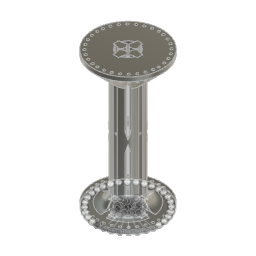
electrically_isolated_longerversion v13 (Autodesk Fusion 360 design; units mm, degrees)
Autodesk Fusion 360 part; units mm, degrees
sketch "Sketch1" plane through (0, 0, 0) normal (0, 0, 1) x (1, 0, 0)
  circle A0 centre (0, 0) radius 10
  circle A1 centre (0, 0) radius 2 construction
  line L0 (-10, 0) -> (10, 0) construction
  line L1 (-10, 0) -> (10, 0) construction
  line L2 (0, 10) -> (0, -10) construction
  line L3 (2, 0) -> (2, 9.798) construction
  line L4 (3.8, 3.2311) -> (3.8, -3.231) construction
  line L5 (3.8, 9.2499) -> (3.8, 0) construction
  spline S0 degree 5 poles (3.8, 3.2311) (3.6635, 3.1018) (3.4023, 2.8433) (3.0464, 2.4556) (2.6446, 1.9386) (2.2717, 1.2924) (2.0398, 0.6462) (1.9604, 0) (2.0398, -0.6462) (2.2717, -1.2924) (2.6446, -1.9386) (3.0464, -2.4556) (3.4023, -2.8433) (3.6635, -3.1018) (3.8, -3.231) knots 0 0 0 0 0 0 0.1 0.2 0.3 0.4 0.5 0.6 0.7 0.8 0.9 1 1 1 1 1 1
  line L6 (7.8, 2) -> (7.8, -2)
  line L7 (5.3, 2.5) -> (5.3, -2.5) construction
  line L8 (5.3, 8.48) -> (5.3, -8.48) construction
  spline S1 degree 5 poles (3.8, 3.2311) (3.8518, 3.1941) (3.9579, 3.1214) (4.1248, 3.0156) (4.3628, 2.8813) (4.6877, 2.7255) (5.0425, 2.5827) (5.4288, 2.4536) (5.8471, 2.3385) (6.2953, 2.2364) (6.7707, 2.1462) (7.1709, 2.0827) (7.4815, 2.0396) (7.6931, 2.0129) (7.8, 2) knots 0 0 0 0 0 0 0.1 0.2 0.3 0.4 0.5 0.6 0.7 0.8 0.9 1 1 1 1 1 1
  spline S2 degree 5 poles (3.8, -3.231) (3.8518, -3.1941) (3.9579, -3.1214) (4.1248, -3.0156) (4.3628, -2.8813) (4.6877, -2.7255) (5.0425, -2.5827) (5.4288, -2.4536) (5.8471, -2.3385) (6.2953, -2.2364) (6.7707, -2.1462) (7.1709, -2.0827) (7.4815, -2.0396) (7.6931, -2.0129) (7.8, -2) knots 0 0 0 0 0 0 0.1 0.2 0.3 0.4 0.5 0.6 0.7 0.8 0.9 1 1 1 1 1 1
  circle A2 centre (0, 0) radius 25
  line L9 (0, -25) -> (0, 25) construction
  circle A3 centre (0, 0) radius 22.5 construction
  circle A4 centre (0, -22.5) radius 0.85
  line L10 (11.8, 2) -> (11.8, -2)
  line L11 (11.8, -2) -> (7.8, -2)
  line L12 (11.8, 2) -> (7.8, 2)
  circle A5 centre (0, 0) radius 7.5
  spline S3 degree 5 poles (-3.2311, 3.8) (-3.1018, 3.6635) (-2.8433, 3.4023) (-2.4556, 3.0464) (-1.9386, 2.6446) (-1.2924, 2.2717) (-0.6462, 2.0398) (0, 1.9604) (0.6462, 2.0398) (1.2924, 2.2717) (1.9386, 2.6446) (2.4556, 3.0464) (2.8433, 3.4023) (3.1018, 3.6635) (3.231, 3.8) knots 0 0 0 0 0 0 0.1 0.2 0.3 0.4 0.5 0.6 0.7 0.8 0.9 1 1 1 1 1 1
  spline S4 degree 5 poles (3.231, 3.8) (3.1941, 3.8518) (3.1214, 3.9579) (3.0156, 4.1248) (2.8813, 4.3628) (2.7255, 4.6877) (2.5827, 5.0425) (2.4536, 5.4288) (2.3385, 5.8471) (2.2364, 6.2953) (2.1462, 6.7707) (2.0827, 7.1709) (2.0396, 7.4815) (2.0129, 7.6931) (2, 7.8) knots 0 0 0 0 0 0 0.1 0.2 0.3 0.4 0.5 0.6 0.7 0.8 0.9 1 1 1 1 1 1
  line L13 (2, 11.8) -> (2, 7.8)
  line L14 (-2, 11.8) -> (2, 11.8)
  line L15 (-2, 7.8) -> (2, 7.8)
  spline S5 degree 5 poles (-3.2311, 3.8) (-3.1941, 3.8518) (-3.1214, 3.9579) (-3.0156, 4.1248) (-2.8813, 4.3628) (-2.7255, 4.6877) (-2.5827, 5.0425) (-2.4536, 5.4288) (-2.3385, 5.8471) (-2.2364, 6.2953) (-2.1462, 6.7707) (-2.0827, 7.1709) (-2.0396, 7.4815) (-2.0129, 7.6931) (-2, 7.8) knots 0 0 0 0 0 0 0.1 0.2 0.3 0.4 0.5 0.6 0.7 0.8 0.9 1 1 1 1 1 1
  line L16 (-2, 11.8) -> (-2, 7.8)
  spline S6 degree 5 poles (-3.8, -3.2311) (-3.6635, -3.1018) (-3.4023, -2.8433) (-3.0464, -2.4556) (-2.6446, -1.9386) (-2.2717, -1.2924) (-2.0398, -0.6462) (-1.9604, 0) (-2.0398, 0.6462) (-2.2717, 1.2924) (-2.6446, 1.9386) (-3.0464, 2.4556) (-3.4023, 2.8433) (-3.6635, 3.1018) (-3.8, 3.231) knots 0 0 0 0 0 0 0.1 0.2 0.3 0.4 0.5 0.6 0.7 0.8 0.9 1 1 1 1 1 1
  spline S7 degree 5 poles (-3.8, 3.231) (-3.8518, 3.1941) (-3.9579, 3.1214) (-4.1248, 3.0156) (-4.3628, 2.8813) (-4.6877, 2.7255) (-5.0425, 2.5827) (-5.4288, 2.4536) (-5.8471, 2.3385) (-6.2953, 2.2364) (-6.7707, 2.1462) (-7.1709, 2.0827) (-7.4815, 2.0396) (-7.6931, 2.0129) (-7.8, 2) knots 0 0 0 0 0 0 0.1 0.2 0.3 0.4 0.5 0.6 0.7 0.8 0.9 1 1 1 1 1 1
  line L17 (-11.8, 2) -> (-7.8, 2)
  line L18 (-11.8, -2) -> (-11.8, 2)
  line L19 (-7.8, -2) -> (-7.8, 2)
  spline S8 degree 5 poles (-3.8, -3.2311) (-3.8518, -3.1941) (-3.9579, -3.1214) (-4.1248, -3.0156) (-4.3628, -2.8813) (-4.6877, -2.7255) (-5.0425, -2.5827) (-5.4288, -2.4536) (-5.8471, -2.3385) (-6.2953, -2.2364) (-6.7707, -2.1462) (-7.1709, -2.0827) (-7.4815, -2.0396) (-7.6931, -2.0129) (-7.8, -2) knots 0 0 0 0 0 0 0.1 0.2 0.3 0.4 0.5 0.6 0.7 0.8 0.9 1 1 1 1 1 1
  line L20 (-11.8, -2) -> (-7.8, -2)
  spline S9 degree 5 poles (3.2311, -3.8) (3.1018, -3.6635) (2.8433, -3.4023) (2.4556, -3.0464) (1.9386, -2.6446) (1.2924, -2.2717) (0.6462, -2.0398) (0, -1.9604) (-0.6462, -2.0398) (-1.2924, -2.2717) (-1.9386, -2.6446) (-2.4556, -3.0464) (-2.8433, -3.4023) (-3.1018, -3.6635) (-3.231, -3.8) knots 0 0 0 0 0 0 0.1 0.2 0.3 0.4 0.5 0.6 0.7 0.8 0.9 1 1 1 1 1 1
  spline S10 degree 5 poles (-3.231, -3.8) (-3.1941, -3.8518) (-3.1214, -3.9579) (-3.0156, -4.1248) (-2.8813, -4.3628) (-2.7255, -4.6877) (-2.5827, -5.0425) (-2.4536, -5.4288) (-2.3385, -5.8471) (-2.2364, -6.2953) (-2.1462, -6.7707) (-2.0827, -7.1709) (-2.0396, -7.4815) (-2.0129, -7.6931) (-2, -7.8) knots 0 0 0 0 0 0 0.1 0.2 0.3 0.4 0.5 0.6 0.7 0.8 0.9 1 1 1 1 1 1
  line L21 (-2, -11.8) -> (-2, -7.8)
  line L22 (2, -11.8) -> (-2, -11.8)
  line L23 (2, -7.8) -> (-2, -7.8)
  spline S11 degree 5 poles (3.2311, -3.8) (3.1941, -3.8518) (3.1214, -3.9579) (3.0156, -4.1248) (2.8813, -4.3628) (2.7255, -4.6877) (2.5827, -5.0425) (2.4536, -5.4288) (2.3385, -5.8471) (2.2364, -6.2953) (2.1462, -6.7707) (2.0827, -7.1709) (2.0396, -7.4815) (2.0129, -7.6931) (2, -7.8) knots 0 0 0 0 0 0 0.1 0.2 0.3 0.4 0.5 0.6 0.7 0.8 0.9 1 1 1 1 1 1
  line L24 (2, -11.8) -> (2, -7.8)
  circle A6 centre (22.5, 0) radius 0.85
  circle A7 centre (0, 22.5) radius 0.85
  circle A8 centre (-22.5, 0) radius 0.85
  circle A9 centre (4.4774, -22.05) radius 0.8625
  circle A10 centre (8.7758, -20.718) radius 0.875
  circle A11 centre (12.7231, -18.5573) radius 0.8875
  circle A12 centre (16.1615, -15.6543) radius 0.9
  circle A13 centre (18.9534, -12.1251) radius 0.9125
  line L25 (0, 0) -> (4.4774, -22.05) construction
  line L26 (0, 0) -> (8.7758, -20.718) construction
  line L27 (0, 0) -> (12.7231, -18.5573) construction
  line L28 (0, 0) -> (16.1615, -15.6543) construction
  line L29 (0, 0) -> (18.9534, -12.1251) construction
  circle A14 centre (20.9872, -8.1109) radius 0.925
  circle A15 centre (22.1815, -3.7723) radius 0.9375
  line L30 (20.9872, -8.1109) -> (0, 0) construction
  line L31 (22.1815, -3.7723) -> (0, 0) construction
  circle A16 centre (22.05, 4.4774) radius 0.8625
  circle A17 centre (20.718, 8.7758) radius 0.875
  circle A18 centre (18.5573, 12.7231) radius 0.8875
  circle A19 centre (15.6543, 16.1615) radius 0.9
  circle A20 centre (12.1251, 18.9534) radius 0.9125
  circle A21 centre (8.1109, 20.9872) radius 0.925
  circle A22 centre (3.7723, 22.1815) radius 0.9375
  circle A23 centre (-4.4774, 22.05) radius 0.8625
  circle A24 centre (-8.7758, 20.718) radius 0.875
  circle A25 centre (-12.7231, 18.5573) radius 0.8875
  circle A26 centre (-16.1615, 15.6543) radius 0.9
  circle A27 centre (-18.9534, 12.1251) radius 0.9125
  circle A28 centre (-20.9872, 8.1109) radius 0.925
  circle A29 centre (-22.1815, 3.7723) radius 0.9375
  circle A30 centre (-22.05, -4.4774) radius 0.8625
  circle A31 centre (-20.718, -8.7758) radius 0.875
  circle A32 centre (-18.5573, -12.7231) radius 0.8875
  circle A33 centre (-15.6543, -16.1615) radius 0.9
  circle A34 centre (-12.1251, -18.9534) radius 0.9125
  circle A35 centre (-8.1109, -20.9872) radius 0.925
  circle A36 centre (-3.7723, -22.1815) radius 0.9375
  line L32 (-8.8, 2) -> (-8.8, -2)
  line L33 (-2, -8.8) -> (2, -8.8)
  line L34 (8.8, -2) -> (8.8, 2)
  line L35 (2, 8.8) -> (-2, 8.8)
  point P0 (5.3, 0)
  point P1 (0, -22.5)
  point P2 (7.8, 0)
  point P3 (0, 2)
  point P4 (2.5, 5.3)
  point P5 (-2.5, 5.3)
  point P6 (-2, 0)
  point P7 (-5.3, 2.5)
  point P8 (-5.3, -2.5)
  point P9 (0, -2)
  point P10 (-2.5, -5.3)
  point P11 (2.5, -5.3)
  dimension "d3" = 20
  dimension "d4" = 4
  dimension "d9" = 1.8
  dimension "d11" = 1.8
  dimension "d12" = 6.4621
  dimension "d16" = 5
  dimension "d17" = 4
  dimension "d18" = 2
  dimension "d19" = 1.5
  dimension "d20" = 50
  dimension "d21" = 45
  dimension "d22" = 1.7
  dimension "d25" = 4
  dimension "d26" = 2.5
  dimension "d28" = 15
  dimension "d31" = 360
  dimension "d33" = 360
  dimension "d102" = 1.725
  dimension "d103" = 1.75
  dimension "d104" = 1.775
  dimension "d105" = 1.8
  dimension "d106" = 1.825
  dimension "d121" = 4.5
  dimension "d123" = 4.5
  dimension "d124" = 4.5
  dimension "d125" = 4.5
  dimension "d126" = 4.5
  dimension "d127" = 4.5
  dimension "d128" = 4.5
  dimension "d129" = 1.85
  dimension "d130" = 1.875
  dimension "d132" = 360
  dimension "d190" = 1
  dimension "d192" = 360
  constraint coincident A0.centre A1.centre
  constraint concentric A0 A1
  constraint coincident A0 L0.start
  constraint coincident A0 L0.end
  constraint horizontal L0
  constraint coincident A0 L2.start
  constraint coincident A0 L2.end
  constraint perpendicular L1 L2
  constraint coincident L1 L3.start
  constraint coincident A1 L3.start
  constraint coincident A0 L3.end
  constraint perpendicular L1 L3
  constraint perpendicular L1 L4
  constraint coincident A0 L5.start
  constraint coincident L0 L5.end
  constraint perpendicular L0 L5
  constraint midpoint L4 L5.end
  constraint vertical L6
  constraint perpendicular L0 L7
  constraint coincident A0 L8.start
  constraint coincident A0 L8.end
  constraint perpendicular L0 L8
  constraint midpoint L8 P0
  constraint midpoint L7 P0
  constraint concentric A0 A2
  constraint coincident A2 L9.start
  constraint coincident A2 L9.end
  constraint vertical L9
  constraint collinear L2 L9
  constraint concentric A2 A3
  constraint coincident L9 P1
  constraint coincident A3 P1
  constraint coincident P1 A4.centre
  constraint midpoint L9 A0.centre
  constraint vertical L10
  constraint coincident L0 P2
  constraint midpoint L6 P2
  constraint horizontal L12
  constraint horizontal L11
  constraint concentric A3 A5
  constraint coincident A3 A9.centre
  constraint coincident A3 A10.centre
  constraint coincident A3 A11.centre
  constraint coincident A3 A12.centre
  constraint coincident A3 A13.centre
  constraint coincident A9.centre L25.end
  constraint coincident A10.centre L26.end
  constraint coincident A11.centre L27.end
  constraint coincident A12.centre L28.end
  constraint coincident A13.centre L29.end
  constraint coincident A3 A14.centre
  constraint coincident A3 A15.centre
  constraint coincident A14.centre L30.start
  constraint coincident A15.centre L31.start
  constraint coincident L20 L32.end
  constraint perpendicular L20 L32
  constraint coincident L17 L32.start
  measures "d3" diameter of A0
  measures "d4" diameter of A1
  measures "d9" distance of L3.start L4
  measures "d11" distance of L3 L5
  measures "d12" distance of L4.start L4.end
  measures "d16" distance of L7.start L7.end
  measures "d17" distance of L6.end L6.start
  measures "d18" horizontal distance of A0.centre L3.start
  measures "d19" distance of L4 L7
  measures "d20" diameter of A2
  measures "d21" diameter of A3
  measures "d22" diameter of A4
  measures "d25" distance of L6 L10
  measures "d26" distance of P0 P2
  measures "d28" diameter of A5
  measures "d102" diameter of A9
  measures "d103" diameter of A10
  measures "d104" diameter of A11
  measures "d105" diameter of A12
  measures "d106" diameter of A13
  measures "d121" distance of P1 A9.centre
  measures "d123" distance of A9.centre A10.centre
  measures "d124" distance of A10.centre A11.centre
  measures "d125" distance of A11.centre A12.centre
  measures "d126" distance of A12.centre A13.centre
  measures "d127" distance of A13.centre A14.centre
  measures "d128" distance of A14.centre A15.centre
  measures "d129" diameter of A14
  measures "d130" diameter of A15
  measures "d190" distance of L19 L32
extrude "Extrude1" add sketch "Sketch1" along normal blind 3 contours A0 L11 L12 L34 | A0 L10 L11 L12 | A0 L13 L16 L35 | A0 L13 L14 L16 | L6 L11 L12 L34 | A0 L21 L22 L24 | A0 L21 L24 L33 | L13 L15 L16 L35 | L21 L23 L24 L33 | A0 L17 L20 L32 | A0 L17 L18 L20 | L17 L19 L20 L32 | A2 | A9 | A10 | A11 | A12 | A13 | A14 | A15 | A16 | A17 | A18 | A19 | A20 | A21 | A22 | A23 | A24 | A25 | A26 | A27 | A28 | A29 | A30 | A31 | A32 | A33 | A34 | A35 | A36 makes body 1
sketch "Sketch2" plane through (0, 0, 3) normal (0, 0, 1) x (-1, 0, 0)
  arc A0 (9.798, 2) -> (2, 9.798) centre (0, 0) ccw
  line L0 (9.798, 2) -> (7.8, 2)
  line L1 (7.8, 2) -> (7.8, -2)
  line L2 (7.8, -2) -> (9.798, -2)
  arc A1 (2, -9.798) -> (9.798, -2) centre (0, 0) ccw
  line L3 (2, -9.798) -> (2, -7.8)
  line L4 (2, -7.8) -> (-2, -7.8)
  line L5 (-2, -7.8) -> (-2, -9.798)
  arc A2 (-9.798, -2) -> (-2, -9.798) centre (0, 0) ccw
  line L6 (-9.798, -2) -> (-7.8, -2)
  line L7 (-7.8, -2) -> (-7.8, 2)
  line L8 (-7.8, 2) -> (-9.798, 2)
  arc A3 (-2, 9.798) -> (-9.798, 2) centre (0, 0) ccw
  line L9 (-2, 9.798) -> (-2, 7.8)
  line L10 (-2, 7.8) -> (2, 7.8)
  line L11 (2, 7.8) -> (2, 9.798)
  circle A4 centre (0, -22.5) radius 0.85
  circle A5 centre (22.5, 0) radius 0.85
  circle A6 centre (0, 22.5) radius 0.85
  circle A7 centre (-22.5, 0) radius 0.85
  circle A8 centre (0, 0) radius 25
  circle A9 centre (0, 0) radius 19.5
  dimension "d36" = 39
  constraint concentric A0 A9
  measures "d36" diameter of A9
extrude "Extrude2" add sketch "Sketch1" along normal blind 100 separate body contours L6 S1 S2 A5 | A5 S4 L15 S5 | S0 S1 S2 A5 | A5 S10 L23 S11 | A5 S3 S4 S5 | A5 S9 S10 S11 | A5 S7 L19 S8 | A5 S6 S7 S8 makes body 2 at (2.4618, 3.0723, 59.5238) makes body 3 at (3.0723, -2.4618, 59.5238) makes body 4 at (-3.0723, 2.4618, 59.5238) makes body 5 at (-2.4618, -3.0723, 59.5238)
copy_body "Body->Comp1" bodies 2 removing the originals makes body 6 in component "rod1"
copy_body "Body->Comp2" bodies 3 removing the originals makes body 7 in component "rod2"
copy_body "Body->Comp3" bodies 4 removing the originals makes body 8 in component "rod3"
copy_body "Body->Comp4" bodies 5 removing the originals makes body 9 in component "rod4"
extrude "Extrude1'" add sketch "Sketch1" along normal blind 100 separate body contours A0 S1 L12 A5 S4 L13 | A0 S2 L11 A5 S11 L24 | A0 A5 S5 L16 S7 L17 | A0 A5 S8 L20 S10 L21 makes body 10 at (-4.3019, 9.0274, 66.6667) makes body 11 at (9.6891, 2.4743, 33.3333) makes body 12 at (-2.4743, -9.6891, 66.6667) makes body 13 at (9.6891, -2.4743, 66.6667) in component "Component"
combine "Combine1" operation add target body 13 tool bodies 12 11 1 10 in component "Component"
fillet "Fillet1" radius 8 1 edges at (-7.0711, -7.0711, 3) on bodies 13 in component "Component"
fillet "Fillet1" radius 8 3 edges at (7.0711, -7.0711, 3) (7.0711, 7.0711, 3) (-7.0711, 7.0711, 3) on bodies 13 in component "Component"
ref_plane "WorkPlane1" through (-5.899, 5.899, 100) normal (0, 0, 1) x (1, 0, 0)
sketch "Sketch3" plane through (-5.8903, 5.8903, 100) normal (0, 0, 1) x (1, 0, 0)
  arc A0 (7.8903, -23.7788) -> (23.7788, -7.8903) centre (5.8903, -5.8903) ccw
  arc A1 (-11.9982, -7.8903) -> (3.8903, -23.7788) centre (5.8903, -5.8903) ccw
  arc A2 (3.8903, 11.9982) -> (-11.9982, -3.8903) centre (5.8903, -5.8903) ccw
  arc A3 (23.7788, -3.8903) -> (7.8903, 11.9982) centre (5.8903, -5.8903) ccw
  point P0 (18.6182, -18.6182)
  point P1 (18.6182, 6.8376)
  point P2 (-6.8376, 6.8376)
  point P3 (-6.8376, -18.6182)
  constraint midpoint A0 P0
  constraint midpoint A3 P1
  constraint midpoint A2 P2
  constraint midpoint A1 P3
ref_plane "WorkPlane2" through (7.0711, -7.0711, 100) normal (0.707107, -0.707107, 0) x (0.707107, 0.707107, 0)
ref_plane "WorkPlane3" through (7.0711, 7.0711, 100) normal (0.707107, 0.707107, 0) x (-0.707107, 0.707107, 0)
ref_plane "WorkPlane4" through (-7.0711, 7.0711, 100) normal (-0.707107, 0.707107, 0) x (-0.707107, -0.707107, 0)
ref_plane "WorkPlane5" through (-7.0711, -7.0711, 100) normal (-0.707107, -0.707107, 0) x (0.707107, -0.707107, 0)
sketch "Sketch4" plane through (7.0711, -7.0711, 100) normal (0.707107, -0.707107, 0) x (0.707107, 0.707107, 0)
  line L0 (25, -100) -> (-25, -100)
  line L1 (-1.6, -89) -> (0, -94.5)
  line L2 (0, -94.5) -> (1.6, -89)
  line L3 (-1.6, -89) -> (1.6, -89) construction
  line L4 (0, 0) -> (0, -100) construction
  line L5 (-1.6, -59) -> (0, -53.5)
  line L6 (0, -53.5) -> (1.6, -59)
  line L7 (-1.6, -59) -> (1.6, -59) construction
  line L8 (0, -83.5) -> (0, -94.5) construction
  line L9 (0, -64.5) -> (0, -53.5) construction
  line L10 (-1.6, -89) -> (-1.6, -59)
  line L11 (1.6, -89) -> (1.6, -59)
  line L12 (0, -50.75) -> (-1.6, -45.25)
  line L13 (-1.6, -45.25) -> (0, -50.75)
  line L14 (0, -50.75) -> (1.6, -45.25)
  line L15 (1.6, -45.25) -> (1.6, -15.25)
  line L16 (1.6, -15.25) -> (0, -9.75)
  line L17 (0, -9.75) -> (-1.6, -15.25)
  line L18 (-1.6, -15.25) -> (-1.6, -45.25)
  line L19 (-1.6, -15.25) -> (1.6, -15.25) construction
  line L20 (-1.6, -45.25) -> (1.6, -45.25) construction
  point P0 (0, -100)
  point P1 (0, -45.25)
  dimension "d52" = 5.5
  dimension "d56" = 3.2
  dimension "d57" = 100
  dimension "d61" = 3.2
  dimension "d147" = 30
  dimension "d148" = 5.5
  dimension "d149" = 5.5
  dimension "d253" = 30
  dimension "d254" = 2.75
  dimension "d256" = 5.5
  dimension "d257" = 5.5
  dimension "d258" = 3.2
  constraint midpoint L0 P0
  constraint horizontal L3
  constraint coincident P0 L4.end
  constraint vertical L4
  constraint coincident L8.start L4
  constraint coincident L1.end L4
  constraint coincident L4 L9.start
  constraint coincident L4 L5.end
  constraint horizontal L7
  constraint midpoint L3 L8
  constraint midpoint L7 L9
  constraint coincident L4 L12.start
  constraint parallel L4 L15
  constraint coincident L4 L16.end
  constraint horizontal L20
  constraint horizontal L19
  constraint parallel L15 L18
  constraint midpoint L20 P1
  constraint coincident L4 P1
  measures "d52" distance of L0 L1.end
  measures "d56" distance of L1.start L2.end
  measures "d57" distance of L0 L4.start
  measures "d61" distance of L5.start L6.end
  measures "d147" distance of L3 L7
  measures "d148" distance of L5.end L7
  measures "d149" distance of L1.end L3
  measures "d253" distance of L19 L20
  measures "d254" distance of L5.end L12.start
  measures "d256" distance of L16.end L19
  measures "d257" distance of L12.start L20
  measures "d258" distance of L15 L18
extrude "Extrude2'" cut sketch "Sketch4" along normal blind -100 and the other way blind -10 bodies 13 in component "Component"
sketch "Sketch5" plane through (-5.8903, 5.8903, 100) normal (0, 0, 1) x (1, 0, 0)
  circle A0 centre (5.8903, -5.8903) radius 25
  circle A1 centre (5.8903, -5.8903) radius 22.5 construction
  line L0 (5.8903, -30.8903) -> (5.8903, 19.1097) construction
  circle A2 centre (5.8903, -5.8903) radius 10
  line L1 (-4.1097, -5.8903) -> (15.8903, -5.8903)
  spline S0 degree 5 poles (2.6592, -2.0903) (2.6962, -2.0385) (2.7689, -1.9324) (2.8747, -1.7655) (3.009, -1.5275) (3.1648, -1.2025) (3.3076, -0.8478) (3.4367, -0.4615) (3.5518, -0.0432) (3.6539, 0.405) (3.7441, 0.8804) (3.8076, 1.2806) (3.8507, 1.5912) (3.8774, 1.8028) (3.8903, 1.9097) knots 0 0 0 0 0 0 0.1 0.2 0.3 0.4 0.5 0.6 0.7 0.8 0.9 1 1 1 1 1 1
  spline S1 degree 5 poles (2.6592, -2.0903) (2.7885, -2.2268) (3.047, -2.4879) (3.4347, -2.8439) (3.9517, -3.2457) (4.5979, -3.6186) (5.2441, -3.8505) (5.8903, -3.9299) (6.5365, -3.8505) (7.1827, -3.6186) (7.8289, -3.2457) (8.3459, -2.8439) (8.7336, -2.4879) (8.9921, -2.2268) (9.1213, -2.0903) knots 0 0 0 0 0 0 0.1 0.2 0.3 0.4 0.5 0.6 0.7 0.8 0.9 1 1 1 1 1 1
  spline S2 degree 5 poles (2.0903, -9.1213) (2.2268, -8.9921) (2.4879, -8.7336) (2.8439, -8.3459) (3.2457, -7.8289) (3.6186, -7.1827) (3.8505, -6.5365) (3.9299, -5.8903) (3.8505, -5.2441) (3.6186, -4.5979) (3.2457, -3.9517) (2.8439, -3.4347) (2.4879, -3.047) (2.2268, -2.7885) (2.0903, -2.6592) knots 0 0 0 0 0 0 0.1 0.2 0.3 0.4 0.5 0.6 0.7 0.8 0.9 1 1 1 1 1 1
  spline S3 degree 5 poles (9.6903, -2.6592) (9.5538, -2.7885) (9.2926, -3.047) (8.9367, -3.4347) (8.5349, -3.9517) (8.162, -4.5979) (7.9301, -5.2441) (7.8507, -5.8903) (7.9301, -6.5365) (8.162, -7.1827) (8.5349, -7.8289) (8.9367, -8.3459) (9.2926, -8.7336) (9.5538, -8.9921) (9.6903, -9.1213) knots 0 0 0 0 0 0 0.1 0.2 0.3 0.4 0.5 0.6 0.7 0.8 0.9 1 1 1 1 1 1
  circle A3 centre (5.8903, -5.8903) radius 2
  spline S4 degree 5 poles (9.1213, -9.6903) (8.9921, -9.5538) (8.7336, -9.2926) (8.3459, -8.9367) (7.8289, -8.5349) (7.1827, -8.162) (6.5365, -7.9301) (5.8903, -7.8507) (5.2441, -7.9301) (4.5979, -8.162) (3.9517, -8.5349) (3.4347, -8.9367) (3.047, -9.2926) (2.7885, -9.5538) (2.6592, -9.6903) knots 0 0 0 0 0 0 0.1 0.2 0.3 0.4 0.5 0.6 0.7 0.8 0.9 1 1 1 1 1 1
  spline S5 degree 5 poles (2.6592, -9.6903) (2.6962, -9.7421) (2.7689, -9.8482) (2.8747, -10.0151) (3.009, -10.253) (3.1648, -10.578) (3.3076, -10.9327) (3.4367, -11.3191) (3.5518, -11.7374) (3.6539, -12.1856) (3.7441, -12.661) (3.8076, -13.0612) (3.8507, -13.3718) (3.8774, -13.5834) (3.8903, -13.6903) knots 0 0 0 0 0 0 0.1 0.2 0.3 0.4 0.5 0.6 0.7 0.8 0.9 1 1 1 1 1 1
  line L2 (3.8903, -17.6903) -> (3.8903, -13.6903)
  line L3 (7.8903, -17.6903) -> (3.8903, -17.6903)
  line L4 (7.8903, -17.6903) -> (7.8903, -13.6903)
  spline S6 degree 5 poles (9.1213, -9.6903) (9.0844, -9.7421) (9.0117, -9.8482) (8.9059, -10.0151) (8.7716, -10.253) (8.6158, -10.578) (8.4729, -10.9327) (8.3439, -11.3191) (8.2288, -11.7374) (8.1267, -12.1856) (8.0365, -12.661) (7.973, -13.0612) (7.9299, -13.3718) (7.9032, -13.5834) (7.8903, -13.6903) knots 0 0 0 0 0 0 0.1 0.2 0.3 0.4 0.5 0.6 0.7 0.8 0.9 1 1 1 1 1 1
  circle A4 centre (5.8903, -5.8903) radius 7.5
  spline S7 degree 5 poles (9.1213, -2.0903) (9.0844, -2.0385) (9.0117, -1.9324) (8.9059, -1.7655) (8.7716, -1.5275) (8.6158, -1.2025) (8.4729, -0.8478) (8.3439, -0.4615) (8.2288, -0.0432) (8.1267, 0.405) (8.0365, 0.8804) (7.973, 1.2806) (7.9299, 1.5912) (7.9032, 1.8028) (7.8903, 1.9097) knots 0 0 0 0 0 0 0.1 0.2 0.3 0.4 0.5 0.6 0.7 0.8 0.9 1 1 1 1 1 1
  line L5 (3.8903, 5.9097) -> (7.8903, 5.9097)
  line L6 (3.8903, 5.9097) -> (3.8903, 1.9097)
  line L7 (3.8903, 1.9097) -> (7.8903, 1.9097)
  line L8 (7.8903, 5.9097) -> (7.8903, 1.9097)
  line L9 (-5.9097, -3.8903) -> (-1.9097, -3.8903)
  spline S8 degree 5 poles (2.0903, -2.6592) (2.0385, -2.6962) (1.9324, -2.7689) (1.7655, -2.8747) (1.5275, -3.009) (1.2025, -3.1648) (0.8478, -3.3076) (0.4615, -3.4367) (0.0432, -3.5518) (-0.405, -3.6539) (-0.8804, -3.7441) (-1.2806, -3.8076) (-1.5912, -3.8507) (-1.8028, -3.8774) (-1.9097, -3.8903) knots 0 0 0 0 0 0 0.1 0.2 0.3 0.4 0.5 0.6 0.7 0.8 0.9 1 1 1 1 1 1
  spline S9 degree 5 poles (2.0903, -9.1213) (2.0385, -9.0844) (1.9324, -9.0117) (1.7655, -8.9059) (1.5275, -8.7716) (1.2025, -8.6158) (0.8478, -8.4729) (0.4615, -8.3439) (0.0432, -8.2288) (-0.405, -8.1267) (-0.8804, -8.0365) (-1.2806, -7.973) (-1.5912, -7.9299) (-1.8028, -7.9032) (-1.9097, -7.8903) knots 0 0 0 0 0 0 0.1 0.2 0.3 0.4 0.5 0.6 0.7 0.8 0.9 1 1 1 1 1 1
  line L10 (-5.9097, -7.8903) -> (-1.9097, -7.8903)
  line L11 (-5.9097, -7.8903) -> (-5.9097, -3.8903)
  line L12 (-1.9097, -7.8903) -> (-1.9097, -3.8903)
  spline S10 degree 5 poles (9.6903, -2.6592) (9.7421, -2.6962) (9.8482, -2.7689) (10.0151, -2.8747) (10.253, -3.009) (10.578, -3.1648) (10.9327, -3.3076) (11.3191, -3.4367) (11.7374, -3.5518) (12.1856, -3.6539) (12.661, -3.7441) (13.0612, -3.8076) (13.3718, -3.8507) (13.5834, -3.8774) (13.6903, -3.8903) knots 0 0 0 0 0 0 0.1 0.2 0.3 0.4 0.5 0.6 0.7 0.8 0.9 1 1 1 1 1 1
  spline S11 degree 5 poles (9.6903, -9.1213) (9.7421, -9.0844) (9.8482, -9.0117) (10.0151, -8.9059) (10.253, -8.7716) (10.578, -8.6158) (10.9327, -8.4729) (11.3191, -8.3439) (11.7374, -8.2288) (12.1856, -8.1267) (12.661, -8.0365) (13.0612, -7.973) (13.3718, -7.9299) (13.5834, -7.9032) (13.6903, -7.8903) knots 0 0 0 0 0 0 0.1 0.2 0.3 0.4 0.5 0.6 0.7 0.8 0.9 1 1 1 1 1 1
  line L13 (17.6903, -7.8903) -> (13.6903, -7.8903)
  line L14 (17.6903, -3.8903) -> (13.6903, -3.8903)
  line L15 (13.6903, -3.8903) -> (13.6903, -7.8903)
  line L16 (17.6903, -3.8903) -> (17.6903, -7.8903)
  line L17 (7.8903, -13.6903) -> (3.8903, -13.6903)
  line L18 (9.6903, -2.6592) -> (9.6903, -9.1213)
  line L19 (11.1903, 2.5897) -> (11.1903, -14.3703)
  line L20 (7.8903, -5.8903) -> (7.8903, 3.9077)
  circle A5 centre (5.8903, -28.3903) radius 0.8
  circle A6 centre (-16.6097, -5.8903) radius 0.8
  circle A7 centre (28.3903, -5.8903) radius 0.8
  circle A8 centre (5.8903, 16.6097) radius 0.8
  point P0 (5.8903, 16.6097)
  point P1 (-16.6097, -5.8903)
  point P2 (5.8903, -28.3903)
  point P3 (28.3903, -5.8903)
  point P4 (11.1903, -14.3703)
  point P5 (5.8903, -7.8903)
  point P6 (8.3903, -11.1903)
  point P7 (11.1903, -3.3903)
  point P8 (11.1903, -8.3903)
  dimension "d77" = 1.6
  dimension "d78" = 1.6
  dimension "d79" = 1.6
  dimension "d80" = 1.6
  constraint coincident P2 A5.centre
  constraint coincident P1 A6.centre
  constraint coincident P3 A7.centre
  constraint coincident P0 A8.centre
  measures "d77" diameter of A5
  measures "d78" diameter of A6
  measures "d79" diameter of A7
  measures "d80" diameter of A8
sketch "Sketch6" plane through (-7.0711, -7.0711, 100) normal (-0.707107, -0.707107, 0) x (0.707107, -0.707107, 0)
  line L0 (25, -100) -> (-25, -100)
  line L1 (0, -100) -> (0, 0) construction
  line L2 (0, -94.5) -> (-1.6, -89)
  line L3 (1.6, -89) -> (0, -94.5)
  line L4 (-1.6, -59) -> (0, -53.5)
  line L5 (0, -53.5) -> (1.6, -59)
  line L6 (0, -53.5) -> (0, -64.5) construction
  line L7 (-1.6, -59) -> (1.6, -59) construction
  line L8 (-1.6, -89) -> (1.6, -89) construction
  line L9 (0, -83.5) -> (0, -94.5) construction
  line L10 (1.6, -89) -> (1.6, -59)
  line L11 (-1.6, -59) -> (-1.6, -89)
  line L12 (0, -50.75) -> (-1.6, -45.25)
  line L13 (-1.6, -45.25) -> (-1.6, -15.25)
  line L14 (-1.6, -15.25) -> (0, -9.75)
  line L15 (0, -9.75) -> (1.6, -15.25)
  line L16 (1.6, -45.25) -> (0, -50.75)
  line L17 (-1.6, -45.25) -> (1.6, -45.25) construction
  line L18 (-1.6, -15.25) -> (1.6, -15.25) construction
  line L19 (1.6, -45.25) -> (1.6, -15.25)
  point P0 (0, -100)
  point P1 (0, -45.25)
  dimension "d62" = 100
  dimension "d63" = 5.5
  dimension "d67" = 3.2
  dimension "d150" = 5.5
  dimension "d151" = 5.5
  dimension "d152" = 30
  dimension "d259" = 2.75
  dimension "d260" = 3.2
  dimension "d261" = 5.5
  dimension "d262" = 5.5
  dimension "d263" = 30
  constraint midpoint L0 P0
  constraint coincident P0 L1.start
  constraint perpendicular L0 L1
  constraint coincident L1 L2.start
  constraint coincident L1 L9.start
  constraint coincident L1 L6.end
  constraint coincident L1 L4.end
  constraint perpendicular L6 L7
  constraint parallel L7 L8
  constraint midpoint L8 L9
  constraint midpoint L6 L7
  constraint perpendicular L7 L10
  constraint coincident L1 L12.start
  constraint coincident L1 L14.end
  constraint midpoint L17 P1
  constraint vertical L13
  constraint vertical L19
  constraint horizontal L17
  constraint horizontal L18
  constraint coincident L1 P1
  measures "d62" distance of P0 L1.end
  measures "d63" distance of P0 L2.start
  measures "d67" distance of L2.end L3.start
  measures "d150" distance of L2.start L8
  measures "d151" distance of L4.end L7
  measures "d152" distance of L7 L8
  measures "d259" distance of L4.end L12.start
  measures "d260" distance of L13 L19
  measures "d261" distance of L12.start L17
  measures "d262" distance of L14.end L18
  measures "d263" distance of L17 L18
extrude "Extrude3" cut sketch "Sketch6" along normal blind -100 and the other way blind -5 bodies 13 in component "Component"
extrude "Extrude4" add sketch "Sketch5" against normal blind 3 contours A0 | A2 L6 L7 L8 L20 | A2 L5 L6 L8 | A2 L13 L14 L16 | A2 L1 L14 L15 | A2 L1 L13 L15 | A2 L1 L9 L12 | A2 L9 L10 L11 | A2 L1 L10 L12 | A2 L2 L3 L4 | A2 L2 L4 L17 | A5 | A6 | A7 | A8 bodies 13 in component "Component"
chamfer "Chamfer1" distance 15 angle 45 1 edges at (-7.0711, 7.0711, 97) on bodies 13 in component "Component"
chamfer "Chamfer1" distance 15 angle 45 3 edges at (-7.0711, -7.0711, 97) (7.0711, -7.0711, 97) (7.0711, 7.0711, 97) on bodies 13 in component "Component"
combine "Combine1'" operation add target body 7 tool bodies 6 9 8 13 in component "rod2"
extrude "Extrude2''" cut sketch "Sketch5" against normal blind 100 contours S0 A4 L7 L20 | L1 A4 S10 L15 | L1 A4 S10 L19 | S1 A4 S7 L20 | L1 S10 L18 L19 | S0 S1 A4 L20 | L1 A4 S11 L15 | L1 A4 S11 L19 | L1 S3 L18 | L1 S11 L18 L19 | L1 A4 S8 L12 | L1 S3 L18 | L1 A4 S9 L12 | L1 S2 A4 S8 | L1 S2 A4 S9 | S4 S5 S6 A4 | S5 S6 A4 L17 bodies 7 in component "rod2"
extrude "Extrude1''" add sketch "Sketch5" against normal blind 100 separate body contours S0 A4 L7 L20 | A4 S7 L20 | L1 A4 S10 L15 | L1 A4 S10 L19 | S1 A4 S7 L20 | L1 S10 L18 L19 | S0 S1 A4 L20 | L1 A4 S11 L15 | L1 A4 S11 L19 | L1 S3 L18 | L1 S11 L18 L19 | L1 A4 S8 L12 | L1 S3 L18 | L1 A4 S9 L12 | L1 S2 A4 S8 | L1 S2 A4 S9 | S4 S5 S6 A4 | S5 S6 A4 L17 makes body 14 at (-7.8, -0.6667, 66.6667) makes body 15 at (-0.6667, 7.8, 66.6667) makes body 16 at (0.6667, -7.8, 66.6667) makes body 17 at (7.8, 0.6667, 66.6667) in component "Component'"
ref_plane "WorkPlane6" through (-17.6777, 17.6777, 1.5) normal (-0.707107, 0.707107, 0) x (-0.707107, -0.707107, 0)
sketch "Sketch7" plane through (-17.6777, 17.6777, 2) normal (-0.707107, 0.707107, 0) x (0.707107, 0.707107, 0)
  circle A0 centre (0, 0) radius 0.8
  dimension "d94" = 1.6
  constraint coincident A0.centre origin
  measures "d94" diameter of A0
extrude "Extrude3'" cut sketch "Sketch7" against normal blind 15 bodies 7 in component "rod2"
pattern_circular "C-Pattern1" count 4 over 360 about axis through (0, 0, 1.75) along (0, 0, 1) of "Extrude3'" in component "rod2"
extrude "Extrude2'''" cut sketch "Sketch1" along normal blind 1.6 contours L6 S1 S2 A5 | A5 S4 L15 S5 | S0 S1 S2 A5 | A5 S10 L23 S11 | A5 S3 S4 S5 | A5 S9 S10 S11 | A5 S7 L19 S8 | A5 S6 S7 S8 bodies 14 15 16 17 in component "Component'"
extrude "Extrude6" add sketch "Sketch1" along normal blind 1.6 contours L6 S1 S2 A5 | A5 S4 L15 S5 | S0 S1 S2 A5 | A5 S10 L23 S11 | A5 S3 S4 S5 | A5 S9 S10 S11 | A5 S7 L19 S8 | A5 S6 S7 S8 bodies 7 in component "rod2"
extrude "Extrude9" add sketch "Sketch5" against normal blind 3 contours A2 L6 L7 L8 L20 bodies 7 in component "rod2"
extrude "Extrude10" add 4 faces at (-0.044, -4.1114, 1.6) (-4.1114, 0.044, 1.6) (0.044, 4.1114, 1.6) (4.1114, -0.044, 1.6) along direction (0, 0, 1) blind 100 on bodies 7 bodies 7 in component "rod2"
extrude "Extrude11" cut 4 faces at (-0.044, -4.1114, 101.6) (-4.1114, 0.044, 101.6) (0.044, 4.1114, 101.6) (4.1114, -0.044, 101.6) along direction (0, 0, -1) blind 100 on bodies 7 bodies 7 in component "rod2"
extrude "Extrude12" add sketch "Sketch1" along normal blind 1.6 contours A0 L13 L16 L35 | A0 L13 L14 L16 | L13 L15 L16 L35 bodies 7 in component "rod2"
sketch "Sketch8" plane through (7.8, 0, 0) normal (1, 0, 0) x (0, 1, 0)
  line L0 (-2, 1.6) -> (2, 1.6)
  line L1 (2, 1.6) -> (2, 100)
  line L2 (2, 100) -> (-2, 100)
  line L3 (-2, 100) -> (-2, 1.6)
  line L4 (-2, 50.8) -> (2, 50.8) construction
  line L5 (0, 1.6) -> (0, 100) construction
  circle A0 centre (0, 50.8) radius 0.7
  dimension "d174" = 1.4
  constraint midpoint L3 L4.start
  constraint midpoint L1 L4.end
  constraint midpoint L0 L5.start
  constraint midpoint L2 L5.end
  constraint midpoint L4 A0.centre
  measures "d174" diameter of A0
extrude "Extrude4'" cut sketch "Sketch8" against normal blind 3.5 contours A0 bodies 17 in component "Component'"
sketch "Sketch9" plane through (0, -7.8, 0) normal (0, -1, 0) x (1, 0, 0)
  line L0 (-2, 1.6) -> (2, 1.6)
  line L1 (2, 1.6) -> (2, 100)
  line L2 (2, 100) -> (-2, 100)
  line L3 (-2, 100) -> (-2, 1.6)
  line L4 (0, 1.6) -> (0, 100) construction
  line L5 (-2, 50.8) -> (2, 50.8) construction
  circle A0 centre (0, 50.8) radius 0.7
  dimension "d181" = 1.4
  constraint midpoint L0 L4.start
  constraint midpoint L2 L4.end
  constraint midpoint L3 L5.start
  constraint midpoint L1 L5.end
  constraint midpoint L4 A0.centre
  measures "d181" diameter of A0
sketch "Sketch10" plane through (0, 7.8, 0) normal (0, 1, 0) x (-1, 0, 0)
  line L0 (-2, 1.6) -> (2, 1.6)
  line L1 (2, 100) -> (-2, 100)
  line L2 (-2, 100) -> (-2, 1.6)
  line L3 (0, 100) -> (0, 1.6) construction
  line L4 (-2, 50.8) -> (2, 50.8) construction
  circle A0 centre (0, 50.8) radius 0.7
  line L5 (2, 1.6) -> (2, 100)
  dimension "d182" = 1.4
  constraint midpoint L1 L3.start
  constraint midpoint L0 L3.end
  constraint midpoint L2 L4.start
  constraint midpoint L4 A0.centre
  measures "d182" diameter of A0
sketch "Sketch11" plane through (-7.8, 0, 0) normal (-1, 0, 0) x (0, -1, 0)
  line L0 (-2, 1.6) -> (2, 1.6)
  line L1 (2, 1.6) -> (2, 100)
  line L2 (2, 100) -> (-2, 100)
  line L3 (-2, 100) -> (-2, 1.6)
  line L4 (0, 100) -> (0, 1.6) construction
  line L5 (-2, 50.8) -> (2, 50.8) construction
  circle A0 centre (0, 50.8) radius 0.7
  dimension "d183" = 1.4
  constraint midpoint L2 L4.start
  constraint midpoint L0 L4.end
  constraint midpoint L3 L5.start
  constraint midpoint L1 L5.end
  constraint midpoint L4 A0.centre
  measures "d183" diameter of A0
extrude "Extrude5" cut sketch "Sketch9" against normal blind 3.5 contours A0 bodies 16 in component "Component'"
extrude "Extrude6'" cut sketch "Sketch10" against normal blind 3.5 contours A0 bodies 15 in component "Component'"
extrude "Extrude7" cut sketch "Sketch11" against normal blind 3.5 contours A0 bodies 14 in component "Component'"
extrude "Extrude13" cut sketch "Sketch1" along normal blind 110 contours L6 L11 L12 L34 | L13 L15 L16 L35 | L21 L23 L24 L33 | L17 L19 L20 L32 bodies 7 in component "rod2"
extrude "Extrude8" add sketch "Sketch1" along normal blind 100 contours L6 L11 L12 L34 | L13 L15 L16 L35 | L21 L23 L24 L33 | L17 L19 L20 L32 bodies 14 15 16 17 in component "Component'"
extrude "Extrude9'" cut sketch "Sketch1" along normal blind 1.6 contours L6 L11 L12 L34 | L13 L15 L16 L35 | L21 L23 L24 L33 | L17 L19 L20 L32 bodies 14 15 16 17 in component "Component'"
extrude "Extrude14" add sketch "Sketch1" along normal blind 1.6 contours L6 L11 L12 L34 | L13 L15 L16 L35 | L21 L23 L24 L33 | L17 L19 L20 L32 bodies 7 in component "rod2"
combine "Combine2" operation add target body 7 tool bodies 17 15 14 16 in component "rod2"
chamfer "Chamfer5" distance 15.99 angle 45 4 edges at (-8.8, 0, 97) (0, -8.8, 97) (8.8, 0, 97) (0, 8.8, 97) on bodies 7 in component "rod2"
extrude "Extrude5'" cut sketch "Sketch1" along normal blind 200 contours A4 | A6 | A7 | A8 | A9 | A10 | A11 | A12 | A13 | A14 | A15 | A16 | A17 | A18 | A19 | A20 | A21 | A22 | A23 | A24 | A25 | A26 | A27 | A28 | A29 | A30 | A31 | A32 | A33 | A34 | A35 | A36 bodies 7 in component "rod2"
extrude "Extrude15" cut sketch "Sketch1" along normal blind 100 contours L6 L11 L12 L34 | L13 L15 L16 L35 | L6 S1 S2 A5 | L21 L23 L24 L33 | A5 S4 L15 S5 | S0 S1 S2 A5 | A5 S10 L23 S11 | L17 L19 L20 L32 | A5 S3 S4 S5 | A5 S9 S10 S11 | A5 S7 L19 S8 | A5 S6 S7 S8 bodies 7 in component "rod2"
extrude "Extrude16" add sketch "Sketch1" along normal blind 1.6 contours L6 L11 L12 L34 | L13 L15 L16 L35 | L6 S1 S2 A5 | L21 L23 L24 L33 | A5 S4 L15 S5 | S0 S1 S2 A5 | A5 S10 L23 S11 | L17 L19 L20 L32 | A5 S3 S4 S5 | A5 S9 S10 S11 | A5 S7 L19 S8 | A5 S6 S7 S8 bodies 7 in component "rod2"
extrude "Extrude17" add 4 faces at (-4.111, 0.0345, 1.6) (-0.0345, -4.111, 1.6) (0.0345, 4.111, 1.6) (4.111, -0.0345, 1.6) along direction (0, 0, 1) blind 98.4 separate body on bodies 7 makes body 18 at (2.4618, 3.0723, 60.1714) makes body 19 at (-3.0723, 2.4618, 60.1714) makes body 20 at (-2.4618, -3.0723, 60.1714) makes body 21 at (3.0723, -2.4618, 60.1714) in component "rod2"
extrude "Extrude3''" add sketch "Sketch1" along normal blind 100 separate body contours L6 L11 L12 L34 | L13 L15 L16 L35 | L6 S1 S2 A5 | L21 L23 L24 L33 | A5 S4 L15 S5 | S0 S1 S2 A5 | A5 S10 L23 S11 | L17 L19 L20 L32 | A5 S3 S4 S5 | A5 S9 S10 S11 | A5 S7 L19 S8 | A5 S6 S7 S8 makes body 22 at (2.4618, 3.0723, 59.5238) makes body 23 at (3.0723, -2.4618, 59.5238) makes body 24 at (-3.0723, 2.4618, 59.5238) makes body 25 at (-2.4618, -3.0723, 59.5238)
copy_body "Body->Comp6" bodies 22 removing the originals makes body 26 in component "Component''"
copy_body "Body->Comp7" bodies 23 removing the originals makes body 27 in component "Component'''"
copy_body "Body->Comp8" bodies 24 removing the originals makes body 28 in component "Component''''"
copy_body "Body->Comp9" bodies 25 removing the originals makes body 29 in component "Component'''''"
extrude "Extrude1'''" cut sketch "Sketch1" along normal blind 1.6 contours L6 L11 L12 L34 | L13 L15 L16 L35 | L6 S1 S2 A5 | L21 L23 L24 L33 | A5 S4 L15 S5 | S0 S1 S2 A5 | A5 S10 L23 S11 | L17 L19 L20 L32 | A5 S3 S4 S5 | A5 S9 S10 S11 | A5 S7 L19 S8 | A5 S6 S7 S8 bodies 26 in component "Component''"
extrude "Extrude1''''" cut sketch "Sketch1" along normal blind 1.6 contours L6 L11 L12 L34 | L13 L15 L16 L35 | L6 S1 S2 A5 | L21 L23 L24 L33 | A5 S4 L15 S5 | S0 S1 S2 A5 | A5 S10 L23 S11 | L17 L19 L20 L32 | A5 S3 S4 S5 | A5 S9 S10 S11 | A5 S7 L19 S8 | A5 S6 S7 S8 bodies 27 in component "Component'''"
extrude "Extrude1'''''" cut sketch "Sketch1" along normal blind 1.6 contours L6 L11 L12 L34 | L13 L15 L16 L35 | L6 S1 S2 A5 | L21 L23 L24 L33 | A5 S4 L15 S5 | S0 S1 S2 A5 | A5 S10 L23 S11 | L17 L19 L20 L32 | A5 S3 S4 S5 | A5 S9 S10 S11 | A5 S7 L19 S8 | A5 S6 S7 S8 bodies 28 in component "Component''''"
extrude "Extrude1''''''" cut sketch "Sketch1" along normal blind 1.6 contours L6 L11 L12 L34 | L13 L15 L16 L35 | L6 S1 S2 A5 | L21 L23 L24 L33 | A5 S4 L15 S5 | S0 S1 S2 A5 | A5 S10 L23 S11 | L17 L19 L20 L32 | A5 S3 S4 S5 | A5 S9 S10 S11 | A5 S7 L19 S8 | A5 S6 S7 S8 bodies 29 in component "Component'''''"
extrude "Extrude18" cut 4 faces at (-0.0345, -4.111, 100) (-4.111, 0.0345, 100) (0.0345, 4.111, 100) (4.111, -0.0345, 100) along direction (0, 0, -1) blind 100 on bodies 18 19 20 21 bodies 7 18 19 20 21 in component "rod2"
extrude "Extrude19" add sketch "Sketch1" along normal blind 1.6 contours L6 L11 L12 L34 | L13 L15 L16 L35 | L6 S1 S2 A5 | L21 L23 L24 L33 | A5 S4 L15 S5 | S0 S1 S2 A5 | A5 S10 L23 S11 | L17 L19 L20 L32 | A5 S3 S4 S5 | A5 S9 S10 S11 | A5 S7 L19 S8 | A5 S6 S7 S8 bodies 7 18 19 20 21 in component "rod2"
extrude "Extrude2''''" [suppressed] in component "Component'''"
extrude "Extrude2'''''" cut sketch "Sketch11" along normal blind 1 and the other way blind 3 contours A0 bodies 28 in component "Component''''"
extrude "Extrude2''''''" cut sketch "Sketch10" along normal blind 1 and the other way blind 3 contours A0 bodies 26 in component "Component''"
extrude "Extrude2'''''''" cut sketch "Sketch9" along normal blind 1 and the other way blind 3 contours A0 bodies 29 in component "Component'''''"
extrude "Extrude3'''" cut sketch "Sketch8" along normal blind 1 and the other way blind 3 contours A0 bodies 27 in component "Component'''"
fillet "Fillet1'" radius 0.5 2 edges at (3.231, 3.8, 50.8) (-3.2311, 3.8, 50.8) on bodies 26 in component "Component''"
fillet "Fillet1''" radius 0.5 2 edges at (3.8, -3.231, 50.8) (3.8, 3.2311, 50.8) on bodies 27 in component "Component'''"
fillet "Fillet1'''" radius 0.5 2 edges at (-3.8, 3.231, 50.8) (-3.8, -3.2311, 50.8) on bodies 28 in component "Component''''"
fillet "Fillet1''''" radius 0.5 2 edges at (3.2311, -3.8, 50.8) (-3.231, -3.8, 50.8) on bodies 29 in component "Component'''''"
fillet "Fillet1'''''" radius 0.5 8 edges at (3.8, 3.2311, 0.8) (3.231, 3.8, 0.8) (3.8, -3.231, 0.8) (3.2311, -3.8, 0.8) (-3.231, -3.8, 0.8) (-3.8, -3.2311, 0.8) (-3.8, 3.231, 0.8) (-3.2311, 3.8, 0.8) on bodies 7 in component "rod2"
component "Component" placed x (1, 0, 0) y (0, 1, 0) z (0, 0, 1) at (0, 0, 0)
component "Component'" placed x (1, 0, 0) y (0, 1, 0) z (0, 0, 1) at (0, 0, 0)
component "rod1" placed x (1, 0, 0) y (0, 1, 0) z (0, 0, 1) at (0, 0, 0)
component "rod2" placed x (1, 0, 0) y (0, 1, 0) z (0, 0, 1) at (0, 0, 0)
component "rod3" placed x (1, 0, 0) y (0, 1, 0) z (0, 0, 1) at (0, 0, 0)
component "rod4" placed x (1, 0, 0) y (0, 1, 0) z (0, 0, 1) at (0, 0, 0)
component "Component'" placed x (1, 0, 0) y (0, 1, 0) z (0, 0, 1) at (0, 0, 0)
component "Component''" placed x (1, 0, 0) y (0, 1, 0) z (0, 0, 1) at (0, 0, 0)
component "Component'''" placed x (1, 0, 0) y (0, 1, 0) z (0, 0, 1) at (0, 0, 0)
component "Component''''" placed x (1, 0, 0) y (0, 1, 0) z (0, 0, 1) at (0, 0, 0)
component "Component'''''" placed x (1, 0, 0) y (0, 1, 0) z (0, 0, 1) at (0, 0, 0)
equation "r0 = 2 mm"
equation "quadrupole_diameter = 20 mm"
equation "d3 = quadrupole_diameter"
equation "d4 = r0 * 2"
equation "parabolic_width = 6.4621 mm"
equation "parabolic_height = 1.8 mm"
equation "d9 = parabolic_height"
equation "d11 = parabolic_height"
equation "d12 = parabolic_width"
equation "rod_length = 10 mm"
equation "d16 = r0 * 2.5"
equation "d17 = r0 * 2"
equation "d18 = r0"
equation "d19 = r0 * 0.75"
equation "d21 = outer_circle_diameter"
equation "diameter_outer_holes = 1.6 mm"
equation "outer_circle_diameter = 45 mm"
equation "quadrupole_inner_diameter = 15 mm"
equation "d28 = quadrupole_inner_diameter"
equation "d34 = baseplate_height"
equation "d36 = attachment_point_slope_start"
equation "attachment_point_slope_start = 39 mm"
equation "height = 100 mm"
equation "d39 = height"
equation "d41 = height"
equation "d44 = fillet_length"
equation "fillet_length = 8 mm"
equation "d47 = fillet_length"
equation "diamond_height = 30 mm"
equation "diamond_width = 3.2 mm"
equation "d52 = diamond_spacing"
equation "d56 = diamond_width"
equation "d57 = height"
equation "diamond_spacing = 5.5 mm"
equation "d61 = diamond_width"
equation "d62 = height"
equation "d63 = diamond_spacing"
equation "d67 = diamond_width"
equation "baseplate_height = 3 mm"
equation "d73 = -baseplate_height"
equation "d77 = diameter_outer_holes"
equation "d78 = diameter_outer_holes"
equation "d79 = diameter_outer_holes"
equation "d80 = diameter_outer_holes"
equation "d83 = ( outer_circle_diameter - quadrupole_inner_diameter ) / 2"
equation "d84 = ( outer_circle_diameter - quadrupole_inner_diameter ) / 2"
equation "chamfer_distance = 15 mm + 0.7979 mm"
equation "d89 = -height"
equation "d91 = -height"
equation "d94 = diameter_outer_holes"
equation "d121 = hole_spacing"
equation "hole_spacing = 4.5 mm"
equation "d123 = hole_spacing"
equation "d124 = hole_spacing"
equation "d125 = hole_spacing"
equation "d126 = hole_spacing"
equation "d127 = hole_spacing"
equation "d128 = hole_spacing"
equation "quadrupolerods_fillet = 0.4 mm"
equation "pla_bottom_conductive_base = 1.6 mm"
equation "d141 = pla_bottom_conductive_base"
equation "d143 = pla_bottom_conductive_base"
equation "d147 = diamond_height"
equation "d148 = diamond_spacing"
equation "d149 = diamond_spacing"
equation "d150 = diamond_spacing"
equation "d151 = diamond_spacing"
equation "d152 = diamond_height"
equation "d162 = -baseplate_height"
equation "d164 = height"
equation "d168 = -height"
equation "d172 = pla_bottom_conductive_base"
equation "d174 = wire_diam"
equation "wire_depth = 3.5 mm"
equation "wire_diam = 1.4 mm"
equation "d181 = wire_diam"
equation "d182 = wire_diam"
equation "d183 = wire_diam"
equation "d184 = -wire_depth"
equation "d186 = -wire_depth"
equation "d188 = -wire_depth"
equation "d193 = height + 10 mm"
equation "d195 = height"
equation "d197 = pla_bottom_conductive_base"
equation "d199 = pla_bottom_conductive_base"
equation "d202 = height"
equation "d204 = pla_bottom_conductive_base"
equation "d206 = height - pla_bottom_conductive_base"
equation "d208 = height"
equation "d210 = pla_bottom_conductive_base"
equation "d212 = pla_bottom_conductive_base"
equation "d214 = pla_bottom_conductive_base"
equation "d216 = pla_bottom_conductive_base"
equation "d218 = -height"
equation "d220 = pla_bottom_conductive_base"
equation "d253 = diamond_height"
equation "d254 = diamond_spacing / 2"
equation "d256 = diamond_spacing"
equation "d257 = diamond_spacing"
equation "d258 = diamond_width"
equation "d259 = diamond_spacing / 2"
equation "d260 = diamond_width"
equation "d261 = diamond_spacing"
equation "d262 = diamond_spacing"
equation "d263 = diamond_height"
